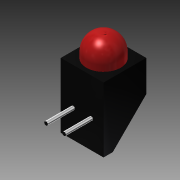
# Autodesk Inventor part: Multicomp-2118128
Saved by Autodesk Inventor 2016 (Build 200138000, 138)
## iProperties
Created: 2017-03-04
Part Number: Multicomp-2118128
Material: Generic
Document SubType Name: Modeling
Designer: Tyler
Density: 1 g/cm^3
Appearance: Glossy - Black
Author: Tyler
Autodesk Inventor part; units mm, degrees
ref_plane "YZ Plane" through (0, 0, 0) normal (1, 0, 0) x (0, 1, 0)
ref_plane "XZ Plane" through (0, 0, 0) normal (0, 1, 0) x (-1, 0, 0)
ref_plane "XY Plane" through (0, 0, 0) normal (0, 0, 1) x (1, 0, 0)
sketch "Sketch1" plane through (0, 0, 0) normal (1, 0, 0) x (0, 1, 0)
  line L0 (0, 5.2) -> (0, -3.9)
  line L1 (0, -3.9) -> (1.3, -3.9)
  line L2 (1.3, -3.9) -> (6, 0.8)
  line L3 (6, 0.8) -> (6, 5.2)
  line L4 (6, 5.2) -> (0, 5.2)
  point P0 (0, 0)
  dimension "d0" = 9.1
  dimension "d1" = 6
  dimension "d2" = 0
  dimension "d3" = 5.2
  dimension "d4" = 1.3
  dimension "d5" = 45
  constraints: 10 end point, 2 perpendicular, 1 parallel, 1 vertical
  measures "d0" distance between parallel lines of L1 L4
  measures "d1" distance of L3.end L0.start
  measures "d2" distance from line of point (0, 0) L0
  measures "d3" distance from line of point (0, 0) L4
  measures "d4" distance of L0.end L1.end
  measures "d5" angle of L3 L2
extrude "Extrusion1" add sketch "Sketch1" along normal mid plane 6
sketch "Sketch2" plane through (-3, 0, 5.2) normal (0, 0, 1) x (1, 0, 0)
  circle A0 centre (3, 3) radius 2.4
  point P0 (3, 0)
  dimension "d8" = 4.8
  constraints: 1 centre point
  measures "d8" diameter of A0
extrude "Extrusion2" add sketch "Sketch2" along normal blind 3.2
fillet "Fillet1" radius 2.4 1 edges at (-2.4, 3, 8.4)
sketch "Sketch3" plane through (-3, 0, -3.9) normal (0, -1, 0) x (1, 0, 0)
  circle A0 centre (1.73, 3.9) radius 0.25
  circle A1 centre (4.27, 3.9) radius 0.25
  point P0 (3, 3.9)
  dimension "d12" = 0.5
  dimension "d13" = 0.5
  dimension "d14" = 2.54
  dimension "d15" = 1.27
  dimension "d16" = 0
  dimension "d17" = 0
  constraints: 2 centre point
  measures "d12" diameter of A0
  measures "d13" diameter of A1
  measures "d14" distance of A1.centre A0.centre
  measures "d15" distance of A0.centre point (3, 3.9)
  measures "d16" vertical distance of A0.centre point (3, 3.9)
  measures "d17" vertical distance of A1.centre point (3, 3.9)
extrude "Extrusion3" add sketch "Sketch3" along normal blind 3.8
equation "\"d15\" = 0.5 * d14"
body "Solid1"
